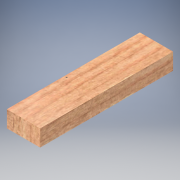
# Autodesk Inventor part: 1x2 Risers
Saved by Autodesk Inventor 2019 (Build 230136000, 136)
## iProperties
Created: 2020-12-30
Part Number: 1x2 Risers
Material: Wood (Birch)
Document SubType Name: Modeling
Designer: John
Density: 0.55 g/cm^3
Appearance: Birch - Natural Polished
Author: John
Autodesk Inventor part; units mm, degrees
ref_plane "YZ Plane" through (0, 0, 0) normal (1, 0, 0) x (0, 1, 0)
ref_plane "XZ Plane" through (0, 0, 0) normal (0, 1, 0) x (-1, 0, 0)
ref_plane "XY Plane" through (0, 0, 0) normal (0, 0, 1) x (1, 0, 0)
sketch "Sketch1" plane through (0, 0, 0) normal (0, 0, 1) x (1, 0, 0)
  line L0 (-19.05, -9.525) -> (19.05, -9.525)
  line L1 (19.05, -9.525) -> (19.05, 9.525)
  line L2 (19.05, 9.525) -> (-19.05, 9.525)
  line L3 (-19.05, 9.525) -> (-19.05, -9.525)
  line L4 (-19.05, -9.525) -> (19.05, 9.525) construction
  line L5 (19.05, -9.525) -> (-19.05, 9.525) construction
  point P0 (0, 0)
  dimension "d0" = 38.1
  dimension "d1" = 19.05
  constraints: 12 end point, 2 midpoint, 2 parallel, 1 horizontal, 1 perpendicular
  measures "d0" distance of L2.end L1.end
  measures "d1" distance of L1.end L0.end
extrude "Extrusion1" add sketch "Sketch1" along normal mid plane 152.4
body "Solid1"
